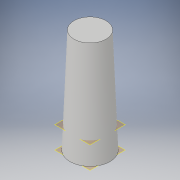
# Autodesk Inventor part: button extension
Saved by Autodesk Inventor 2019 (Build 230136000, 136)
## iProperties
Created: 2020-02-24
Part Number: button extension
Material: Generic
Document SubType Name: Modeling
Designer: close
Density: 1 g/cm^3
Appearance: Default
Author: close
Autodesk Inventor part; units mm, degrees
ref_plane "YZ Plane" through (0, 0, 0) normal (1, 0, 0) x (0, 1, 0)
ref_plane "XY Plane" through (0, 0, 0) normal (0, 0, 1) x (1, 0, 0)
sketch "Sketch1" plane through (0, 0, 0) normal (0, 1, 0) x (-1, 0, 0)
  circle A0 centre (0, 0) radius 2
  dimension "d0" = 4
  constraints: 1 centre point, 1 coincident
  measures "d0" diameter of A0
ref_plane "Work Plane1" through (0, -13, 0) normal (0, 1, 0) x (-1, 0, 0)
sketch "Sketch2" plane through (0, -13, 0) normal (0, 1, 0) x (-1, 0, 0)
  circle A0 centre (0, 0) radius 2.5
  dimension "d2" = 5
  constraints: 1 centre point, 1 coincident
  measures "d2" diameter of A0
ref_plane "Work Plane2" through (0, -10.25, 0) normal (0, 1, 0) x (-1, 0, 0)
sketch "Sketch3" plane through (0, -10.25, 0) normal (0, 1, 0) x (-1, 0, 0)
  circle A0 centre (0, 0) radius 1.65
  dimension "d5" = 3.3
  constraints: 1 centre point, 1 coincident
  measures "d5" diameter of A0
loft "Loft1" add profiles "Sketch1", "Sketch2"
sketch "Sketch5" plane through (0, -13, 0) normal (0, -1, 0) x (1, 0, 0)
  circle A0 centre (0, 0) radius 1.875
  dimension "d10" = 3.75
  constraints: 1 centre point, 1 coincident
  measures "d10" diameter of A0
loft "Loft2" cut profiles "Sketch3", "Sketch5"
body "Solid1"
